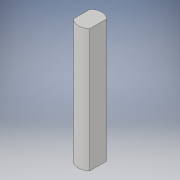
# Autodesk Inventor part: joint_1_os
Saved by Autodesk Inventor 2019 (Build 230136000, 136)
## iProperties
Created: 2019-12-26
Part Number: joint_1_os
Material: Типовые
Document SubType Name: Modeling
Designer: Петров Иван
Density: 1 g/cm^3
Appearance: По умолчанию
Author: Петров Иван
Autodesk Inventor part; units mm, degrees
ref_plane "YZ Plane" through (0, 0, 0) normal (1, 0, 0) x (0, 1, 0)
ref_plane "XZ Plane" through (0, 0, 0) normal (0, 1, 0) x (-1, 0, 0)
ref_plane "XY Plane" through (0, 0, 0) normal (0, 0, 1) x (1, 0, 0)
sketch "Эскиз1" plane through (0, 0, 0) normal (0, 1, 0) x (-1, 0, 0)
  line L0 (-6, -6.0208) -> (-6, 6.0208)
  arc A0 (-6, -6.0208) -> (6, -6.0208) centre (0, 0) ccw
  line L1 (6, 6.0208) -> (6, -6.0208)
  arc A1 (6, 6.0208) -> (-6, 6.0208) centre (0, 0) ccw
  constraints: 4 end point, 4 point on circle, 2 centre point
extrude "Выдавливание1" add sketch "Эскиз1" along normal blind 89
